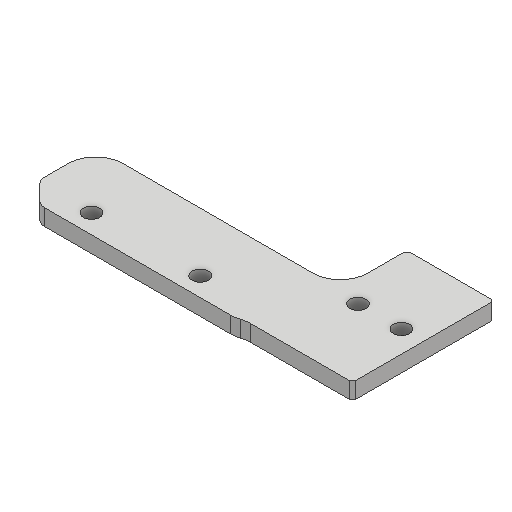
# Autodesk Inventor part: LC_ALU_3mm_Y_Axis_IGUS_Cable_Chain_Mount
Saved by Autodesk Inventor 2026.1 (Build 301233000, 233)
## iProperties
Created: 2016-06-22
Part Number: LC_ALU_3mm_Y_Axis_IGUS_Cable_Chain_Mount
Material: Ogólny
Document SubType Name: Modeling
Designer: Andrzej
Density: 1 g/cm^3
Appearance: Domyślna
Mass: 3.05471 g
Surface Area: 26.5017 cm^2
Volume: 3.05471 cm^3
Author: Andrzej
Autodesk Inventor part; units mm, degrees
ref_plane "YZ Plane" through (0, 0, 0) normal (1, 0, 0) x (0, 1, 0)
ref_plane "XZ Plane" through (0, 0, 0) normal (0, 1, 0) x (-1, 0, 0)
ref_plane "XY Plane" through (0, 0, 0) normal (0, 0, 1) x (1, 0, 0)
sketch "Szkic1" plane through (0, 0, 0) normal (0, 0, 1) x (1, 0, 0)
  line L0 (-15.6232, -1.5262) -> (24.3768, -1.5262)
  line L1 (24.3768, -1.5262) -> (24.3768, -15.7762)
  line L2 (24.3768, -15.7762) -> (-15.6232, -15.7762)
  line L3 (-15.6232, -15.7762) -> (-15.6232, -1.5262)
  line L4 (24.3768, -1.5262) -> (29.3768, -1.5262)
  line L5 (29.3768, -1.5262) -> (29.3768, 10.7238)
  line L6 (29.3768, 10.7238) -> (45.3768, 10.7238)
  line L7 (45.3768, -15.2762) -> (45.3768, 10.7238)
  line L8 (45.3768, -15.2762) -> (24.3768, -15.2762)
  point P0 (0, 0)
  point P1 (-5.6232, -12.2762)
  point P2 (14.3768, -12.2762)
  point P3 (33.3768, -2.2762)
  point P4 (41.3768, -2.2762)
  dimension "d0" = 40
  dimension "d1" = 14.25
  dimension "d2" = 10
  dimension "d3" = 10
  dimension "d4" = 3.5
  dimension "d5" = 3.5
  dimension "d6" = 5
  dimension "d7" = 16
  dimension "d18" = 26
  dimension "d19" = 0.5
  dimension "d20" = 13
  dimension "d21" = 13
  dimension "d22" = 4
  dimension "d23" = 4
  constraints: 18 end point, 4 perpendicular, 3 horizontal, 2 parallel, 1 point on line
  measures "d0" distance of L1.end L2.end
  measures "d1" distance of L0.end L1.end
  measures "d2" distance from line of L3 point (-5.623, -12.276)
  measures "d3" distance from line of L1 point (14.377, -12.276)
  measures "d4" distance from line of L2 point (-5.623, -12.276)
  measures "d5" distance from line of L2 point (14.377, -12.276)
  measures "d6" distance of L0.end L4.end
  measures "d7" distance between parallel lines of L7 L5
  measures "d18" distance of L7.start L6.end
  measures "d19" distance between parallel lines of L2 L8
  measures "d20" distance from line of L8 point (33.377, -2.276)
  measures "d21" distance from line of L8 point (41.377, -2.276)
  measures "d22" distance from line of L5 point (33.377, -2.276)
  measures "d23" distance from line of L7 point (41.377, -2.276)
extrude "Wyciągnięcie proste1" add sketch "Szkic1" along normal blind 3
hole "Otwór1" at (-5.6232, -12.2762, 0) at (14.3768, -12.2762, 0) at (33.3768, -2.2762, 0) at (41.3768, -2.2762, 0) direction (0, 0, 1) diameter 3 end through all
chamfer "Faza1" distance 4 angle 45 1 edges at (-15.6232, -15.7762, 1.5)
fillet "Zaokrąglenie1" radius 2 2 edges at (-15.6232, -11.7762, 1.5) (-11.6232, -15.7762, 1.5)
fillet "Zaokrąglenie2" radius 5 4 edges at (-15.6232, -1.5262, 1.5) (29.3768, -1.5262, 1.5) (24.3768, -15.2762, 1.5) (24.3768, -15.7762, 1.5)
chamfer "Faza2" distance 0.5 angle 45 3 edges at (29.3768, 10.7238, 1.5) (45.3768, 10.7238, 1.5) (45.3768, -15.2762, 1.5)
equation "\"d3\" = d2"
equation "\"d20\" = 0.5 * d18"
equation "\"d21\" = 0.5 * d18"
